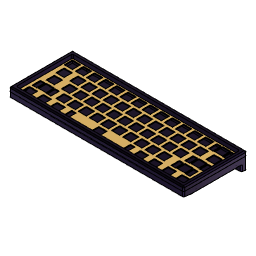
Anatidae60 v9 (Autodesk Fusion 360 design; units mm, degrees)
Autodesk Fusion 360 part; units mm, degrees
note: some values were not read from the file. Chosen so that the rebuilt part matches the saved one: which face or edge a step refers to; that a step has no effect; how an offset face is resized.
(part 1 of 2)
sketch "Sketch1" plane through (0, 0, 0) normal (0, 0, 1) x (1, 0, 0)
  line L0 (193.687761, 24.152837) -> (179.687761, 24.152837)
  line L1 (0.950846, 97.826737) -> (286.700761, 97.826737)
  line L2 (160.637761, 38.152237) -> (174.637761, 38.152237)
  line L3 (196.356761, 5.102877) -> (196.356761, 19.102337)
  line L4 (150.824761, 95.302337) -> (150.824761, 81.303037)
  line L5 (210.355761, 5.102877) -> (196.356761, 5.102877)
  line L6 (124.917761, 9.803347) -> (124.917761, 5.102877)
  line L7 (93.674761, 95.302337) -> (93.674761, 81.303037)
  line L8 (138.918761, 14.401837) -> (138.918761, 19.102337)
  line L9 (67.481061, 19.102337) -> (67.481061, 5.102877)
  line L10 (210.355761, 19.102337) -> (210.355761, 5.102877)
  line L11 (98.437261, 38.152237) -> (98.437261, 24.152837)
  line L12 (43.668561, 19.102337) -> (43.668561, 5.102877)
  line L13 (146.062761, 43.203037) -> (132.062761, 43.203037)
  line L14 (136.537761, 38.152237) -> (136.537761, 24.152837)
  line L15 (51.100461, 62.253037) -> (51.100461, 76.252337)
  line L16 (150.824761, 81.303037) -> (136.825761, 81.303037)
  line L17 (3.475411, 95.302337) -> (17.474961, 95.302337)
  line L18 (10.617791, 43.203037) -> (10.617791, 57.202337)
  line L19 (220.167761, 5.102877) -> (220.167761, 19.102337)
  line L20 (286.700761, 97.826737) -> (286.700761, 2.57693)
  line L21 (46.337961, 38.152237) -> (60.337261, 38.152237)
  line L22 (241.312761, 43.203037) -> (227.312761, 43.203037)
  line L23 (198.737761, 38.152237) -> (212.737761, 38.152237)
  line L24 (79.675461, 95.302337) -> (93.674761, 95.302337)
  line L25 (124.917761, 19.102337) -> (124.917761, 14.401837)
  line L26 (103.487761, 38.152237) -> (117.487761, 38.152237)
  line L27 (243.981761, 5.102877) -> (243.981761, 19.102337)
  line L28 (65.387961, 24.152837) -> (65.387961, 38.152237)
  line L29 (29.381161, 38.152237) -> (15.381661, 38.152237)
  line L30 (113.012761, 57.202337) -> (127.012761, 57.202337)
  line L31 (98.724061, 81.303037) -> (98.724061, 95.302337)
  line L32 (107.962761, 43.203037) -> (93.962961, 43.203037)
  line L33 (41.575461, 81.303037) -> (41.575461, 95.302337)
  line L34 (146.350761, 76.252337) -> (160.349761, 76.252337)
  line L35 (74.624761, 95.302337) -> (74.624761, 81.303037)
  line L36 (122.537761, 24.152837) -> (122.537761, 38.152237)
  line L37 (117.487761, 24.152837) -> (103.487761, 24.152837)
  line L38 (17.474961, 95.302337) -> (17.474961, 81.303037)
  line L39 (79.387261, 24.152837) -> (65.387961, 24.152837)
  line L40 (265.412761, 62.253037) -> (265.412761, 76.252337)
  line L41 (55.574761, 81.303037) -> (41.575461, 81.303037)
  line L42 (55.862961, 43.203037) -> (55.862961, 57.202337)
  line L43 (217.787761, 38.152237) -> (231.787761, 38.152237)
  line L44 (29.667761, 19.102337) -> (43.668561, 19.102337)
  line L45 (132.062761, 43.203037) -> (132.062761, 57.202337)
  line L46 (5.856671, 5.102877) -> (5.856671, 19.102337)
  line L47 (36.812961, 57.202337) -> (50.812261, 57.202337)
  line L48 (138.918761, 19.102337) -> (124.917761, 19.102337)
  line L49 (19.856161, 5.102877) -> (5.856671, 5.102877)
  line L50 (253.505761, 24.152837) -> (267.505761, 24.152837)
  line L51 (8.237921, 76.252337) -> (22.237461, 76.252337)
  line L52 (19.856161, 19.102337) -> (19.856161, 5.102877)
  line L53 (60.337261, 24.152837) -> (46.337961, 24.152837)
  line L54 (53.481761, 19.102337) -> (67.481061, 19.102337)
  line L55 (117.773761, 81.303037) -> (117.773761, 95.302337)
  line L56 (65.387961, 38.152237) -> (79.387261, 38.152237)
  line L57 (88.912261, 57.202337) -> (88.912261, 43.203037)
  line L58 (193.687761, 38.152237) -> (193.687761, 24.152837)
  line L59 (257.980761, 5.102877) -> (243.981761, 5.102877)
  line L60 (174.637761, 24.152837) -> (160.637761, 24.152837)
  line L61 (286.700761, 2.57693) -> (0.950846, 2.57693)
  line L62 (179.687761, 38.152237) -> (193.687761, 38.152237)
  line L63 (43.668561, 5.102877) -> (29.667761, 5.102877)
  line L64 (65.099761, 62.253037) -> (51.100461, 62.253037)
  line L65 (15.381661, 38.152237) -> (15.381661, 33.451837)
  line L66 (8.237921, 62.253037) -> (8.237921, 76.252337)
  line L67 (50.812261, 43.203037) -> (36.812961, 43.203037)
  line L68 (165.112761, 43.203037) -> (151.112761, 43.203037)
  line L69 (131.774761, 81.303037) -> (117.773761, 81.303037)
  line L70 (257.980761, 19.102337) -> (257.980761, 5.102877)
  line L71 (122.537761, 38.152237) -> (136.537761, 38.152237)
  line L72 (117.487761, 38.152237) -> (117.487761, 24.152837)
  line L73 (136.537761, 24.152837) -> (122.537761, 24.152837)
  line L74 (74.912961, 57.202337) -> (88.912261, 57.202337)
  line L75 (281.793761, 5.102877) -> (267.792761, 5.102877)
  line L76 (60.337261, 38.152237) -> (60.337261, 24.152837)
  line L77 (231.787761, 38.152237) -> (231.787761, 24.152837)
  line L78 (70.150461, 62.253037) -> (70.150461, 76.252337)
  line L79 (231.787761, 24.152837) -> (217.787761, 24.152837)
  line L80 (69.862261, 43.203037) -> (55.862961, 43.203037)
  line L81 (107.962761, 57.202337) -> (107.962761, 43.203037)
  line L82 (3.475411, 81.303037) -> (3.475411, 95.302337)
  line L83 (234.168761, 19.102337) -> (234.168761, 5.102877)
  line L84 (267.505761, 38.152237) -> (253.505761, 38.152237)
  line L85 (84.149761, 76.252337) -> (84.149761, 62.253037)
  line L86 (196.356761, 19.102337) -> (210.355761, 19.102337)
  line L87 (29.381161, 24.152837) -> (29.381161, 28.851937)
  line L88 (132.062761, 57.202337) -> (146.062761, 57.202337)
  line L89 (79.675461, 81.303037) -> (79.675461, 95.302337)
  line L90 (198.737761, 24.152837) -> (198.737761, 38.152237)
  line L91 (17.474961, 81.303037) -> (3.475411, 81.303037)
  line L92 (89.200461, 76.252337) -> (103.199761, 76.252337)
  line L93 (127.300761, 62.253037) -> (127.300761, 76.252337)
  line L94 (174.637761, 38.152237) -> (174.637761, 24.152837)
  line L95 (127.300761, 76.252337) -> (141.299761, 76.252337)
  line L96 (212.737761, 24.152837) -> (198.737761, 24.152837)
  line L97 (141.587761, 38.152237) -> (155.587761, 38.152237)
  line L98 (203.212761, 43.203037) -> (189.212761, 43.203037)
  line L99 (67.481061, 5.102877) -> (53.481761, 5.102877)
  line L100 (141.587761, 24.152837) -> (141.587761, 38.152237)
  line L101 (234.168761, 5.102877) -> (220.167761, 5.102877)
  line L102 (179.687761, 24.152837) -> (179.687761, 38.152237)
  line L103 (217.787761, 24.152837) -> (217.787761, 38.152237)
  line L104 (117.773761, 95.302337) -> (131.774761, 95.302337)
  line L105 (222.262761, 43.203037) -> (208.262761, 43.203037)
  line L106 (32.050461, 76.252337) -> (46.049761, 76.252337)
  line L107 (93.962961, 57.202337) -> (107.962761, 57.202337)
  line L108 (103.487761, 24.152837) -> (103.487761, 38.152237)
  line L109 (84.437961, 38.152237) -> (98.437261, 38.152237)
  line L110 (212.737761, 38.152237) -> (212.737761, 24.152837)
  line L111 (127.012761, 57.202337) -> (127.012761, 43.203037)
  line L112 (151.112761, 43.203037) -> (151.112761, 57.202337)
  line L113 (36.524761, 81.303037) -> (22.525461, 81.303037)
  line L114 (36.524761, 95.302337) -> (36.524761, 81.303037)
  line L115 (127.012761, 43.203037) -> (113.012761, 43.203037)
  line L116 (151.112761, 57.202337) -> (165.112761, 57.202337)
  line L117 (50.812261, 57.202337) -> (50.812261, 43.203037)
  line L118 (5.856671, 19.102337) -> (19.856161, 19.102337)
  line L119 (136.825761, 95.302337) -> (150.824761, 95.302337)
  line L120 (53.481761, 5.102877) -> (53.481761, 19.102337)
  line L121 (108.250761, 76.252337) -> (122.249761, 76.252337)
  line L122 (253.505761, 28.851937) -> (253.505761, 24.152837)
  line L123 (60.625461, 95.302337) -> (74.624761, 95.302337)
  line L124 (46.337961, 24.152837) -> (46.337961, 38.152237)
  line L125 (60.625461, 81.303037) -> (60.625461, 95.302337)
  line L126 (15.381661, 24.152837) -> (29.381161, 24.152837)
  line L127 (74.624761, 81.303037) -> (60.625461, 81.303037)
  line L128 (41.575461, 95.302337) -> (55.574761, 95.302337)
  line L129 (122.249761, 62.253037) -> (108.250761, 62.253037)
  line L130 (29.667761, 5.102877) -> (29.667761, 19.102337)
  line L131 (103.199761, 76.252337) -> (103.199761, 62.253037)
  line L132 (220.167761, 19.102337) -> (234.168761, 19.102337)
  line L133 (112.724761, 95.302337) -> (112.724761, 81.303037)
  line L134 (79.387261, 38.152237) -> (79.387261, 24.152837)
  line L135 (88.912261, 43.203037) -> (74.912961, 43.203037)
  line L136 (84.437961, 24.152837) -> (84.437961, 38.152237)
  line L137 (22.525461, 81.303037) -> (22.525461, 95.302337)
  line L138 (138.918761, 5.102877) -> (138.918761, 9.803347)
  line L139 (260.650761, 81.303037) -> (274.649761, 81.303037)
  line L140 (98.437261, 24.152837) -> (84.437961, 24.152837)
  line L141 (55.574761, 95.302337) -> (55.574761, 81.303037)
  line L142 (70.150461, 76.252337) -> (84.149761, 76.252337)
  line L143 (32.050461, 62.253037) -> (32.050461, 76.252337)
  line L144 (22.237461, 76.252337) -> (22.237461, 62.253037)
  line L145 (217.499761, 76.252337) -> (217.499761, 62.253037)
  line L146 (69.862261, 57.202337) -> (69.862261, 43.203037)
  line L147 (255.599761, 62.253037) -> (241.600761, 62.253037)
  line L148 (93.674761, 81.303037) -> (79.675461, 81.303037)
  line L149 (122.249761, 76.252337) -> (122.249761, 62.253037)
  line L150 (281.793761, 19.102337) -> (281.793761, 5.102877)
  line L151 (155.875761, 81.303037) -> (155.875761, 95.302337)
  line L152 (22.237461, 62.253037) -> (8.237921, 62.253037)
  line L153 (131.774761, 95.302337) -> (131.774761, 81.303037)
  line L154 (46.049761, 62.253037) -> (32.050461, 62.253037)
  line L155 (46.049761, 76.252337) -> (46.049761, 62.253037)
  line L156 (89.200461, 62.253037) -> (89.200461, 76.252337)
  line L157 (55.862961, 57.202337) -> (69.862261, 57.202337)
  line L158 (10.617791, 57.202337) -> (24.618661, 57.202337)
  line L159 (103.199761, 62.253037) -> (89.200461, 62.253037)
  line L160 (279.412761, 76.252337) -> (279.412761, 62.253037)
  line L161 (22.525461, 95.302337) -> (36.524761, 95.302337)
  line L162 (141.299761, 62.253037) -> (127.300761, 62.253037)
  line L163 (243.981761, 19.102337) -> (257.980761, 19.102337)
  line L164 (24.618661, 57.202337) -> (24.618661, 43.203037)
  line L165 (74.912961, 43.203037) -> (74.912961, 57.202337)
  line L166 (98.724061, 95.302337) -> (112.724761, 95.302337)
  line L167 (113.012761, 43.203037) -> (113.012761, 57.202337)
  line L168 (155.587761, 24.152837) -> (141.587761, 24.152837)
  line L169 (146.062761, 57.202337) -> (146.062761, 43.203037)
  line L170 (65.099761, 76.252337) -> (65.099761, 62.253037)
  line L171 (24.618661, 43.203037) -> (10.617791, 43.203037)
  line L172 (136.825761, 81.303037) -> (136.825761, 95.302337)
  line L173 (267.505761, 24.152837) -> (267.505761, 28.851937)
  line L174 (36.812961, 43.203037) -> (36.812961, 57.202337)
  line L175 (93.962961, 43.203037) -> (93.962961, 57.202337)
  line L176 (51.100461, 76.252337) -> (65.099761, 76.252337)
  line L177 (170.162761, 57.202337) -> (184.162761, 57.202337)
  line L178 (193.975761, 81.303037) -> (193.975761, 95.302337)
  line L179 (84.149761, 62.253037) -> (70.150461, 62.253037)
  line L180 (160.349761, 76.252337) -> (160.349761, 62.253037)
  line L181 (189.212761, 57.202337) -> (203.212761, 57.202337)
  line L182 (213.025761, 81.303037) -> (213.025761, 95.302337)
  line L183 (203.500761, 62.253037) -> (203.500761, 76.252337)
  line L184 (155.587761, 38.152237) -> (155.587761, 24.152837)
  line L185 (174.925761, 81.303037) -> (174.925761, 95.302337)
  line L186 (267.792761, 5.102877) -> (267.792761, 19.102337)
  line L187 (255.599761, 76.252337) -> (255.599761, 62.253037)
  line L188 (160.637761, 24.152837) -> (160.637761, 38.152237)
  line L189 (108.250761, 62.253037) -> (108.250761, 76.252337)
  line L190 (184.450761, 76.252337) -> (198.449761, 76.252337)
  line L191 (160.349761, 62.253037) -> (146.350761, 62.253037)
  line L192 (267.505761, 33.451837) -> (267.505761, 38.152237)
  line L193 (165.112761, 57.202337) -> (165.112761, 43.203037)
  line L194 (141.299761, 76.252337) -> (141.299761, 62.253037)
  line L195 (267.792761, 19.102337) -> (281.793761, 19.102337)
  line L196 (274.649761, 95.302337) -> (260.650761, 95.302337)
  line L197 (124.917761, 5.102877) -> (138.918761, 5.102877)
  line L198 (232.075761, 95.302337) -> (246.074761, 95.302337)
  line L199 (146.350761, 62.253037) -> (146.350761, 76.252337)
  line L200 (112.724761, 81.303037) -> (98.724061, 81.303037)
  line L201 (227.312761, 43.203037) -> (227.312761, 57.202337)
  line L202 (29.381161, 33.451837) -> (29.381161, 38.152237)
  line L203 (193.975761, 95.302337) -> (207.974761, 95.302337)
  line L204 (272.268761, 57.202337) -> (258.267761, 57.202337)
  line L205 (207.974761, 81.303037) -> (193.975761, 81.303037)
  line L206 (272.268761, 43.203037) -> (272.268761, 47.902037)
  line L207 (165.400761, 62.253037) -> (165.400761, 76.252337)
  line L208 (184.450761, 62.253037) -> (184.450761, 76.252337)
  line L209 (246.074761, 81.303037) -> (232.075761, 81.303037)
  line L210 (15.381661, 28.851937) -> (15.381661, 24.152837)
  line L211 (222.550761, 76.252337) -> (236.549761, 76.252337)
  line L212 (207.974761, 95.302337) -> (207.974761, 81.303037)
  line L213 (253.505761, 38.152237) -> (253.505761, 33.451837)
  line L214 (222.550761, 62.253037) -> (222.550761, 76.252337)
  line L215 (246.074761, 95.302337) -> (246.074761, 81.303037)
  line L216 (274.649761, 90.601837) -> (274.649761, 95.302337)
  line L217 (274.649761, 81.303037) -> (274.649761, 86.002037)
  line L218 (208.262761, 43.203037) -> (208.262761, 57.202337)
  line L219 (179.399761, 62.253037) -> (165.400761, 62.253037)
  line L220 (217.499761, 62.253037) -> (203.500761, 62.253037)
  line L221 (203.212761, 57.202337) -> (203.212761, 43.203037)
  line L222 (227.024761, 81.303037) -> (213.025761, 81.303037)
  line L223 (236.549761, 62.253037) -> (222.550761, 62.253037)
  line L224 (169.874761, 95.302337) -> (169.874761, 81.303037)
  line L225 (227.024761, 95.302337) -> (227.024761, 81.303037)
  line L226 (241.600761, 76.252337) -> (255.599761, 76.252337)
  line L227 (236.549761, 76.252337) -> (236.549761, 62.253037)
  line L228 (232.075761, 81.303037) -> (232.075761, 95.302337)
  line L229 (241.600761, 62.253037) -> (241.600761, 76.252337)
  line L230 (258.267761, 43.203037) -> (272.268761, 43.203037)
  line L231 (188.924761, 81.303037) -> (174.925761, 81.303037)
  line L232 (188.924761, 95.302337) -> (188.924761, 81.303037)
  line L233 (170.162761, 43.203037) -> (170.162761, 57.202337)
  line L234 (179.399761, 76.252337) -> (179.399761, 62.253037)
  line L235 (203.500761, 76.252337) -> (217.499761, 76.252337)
  line L236 (241.312761, 57.202337) -> (241.312761, 43.203037)
  line L237 (169.874761, 81.303037) -> (155.875761, 81.303037)
  line L238 (227.312761, 57.202337) -> (241.312761, 57.202337)
  line L239 (279.412761, 62.253037) -> (265.412761, 62.253037)
  line L240 (222.262761, 57.202337) -> (222.262761, 43.203037)
  line L241 (258.267761, 57.202337) -> (258.267761, 52.501837)
  line L242 (198.449761, 76.252337) -> (198.449761, 62.253037)
  line L243 (208.262761, 57.202337) -> (222.262761, 57.202337)
  line L244 (213.025761, 95.302337) -> (227.024761, 95.302337)
  line L245 (265.412761, 76.252337) -> (279.412761, 76.252337)
  line L246 (272.268761, 52.501837) -> (272.268761, 57.202337)
  line L247 (155.875761, 95.302337) -> (169.874761, 95.302337)
  line L248 (198.449761, 62.253037) -> (184.450761, 62.253037)
  line L249 (258.267761, 47.902037) -> (258.267761, 43.203037)
  line L250 (184.162761, 43.203037) -> (170.162761, 43.203037)
  line L251 (0.950846, 2.57693) -> (0.950846, 97.826737)
  line L252 (184.162761, 57.202337) -> (184.162761, 43.203037)
  line L253 (189.212761, 43.203037) -> (189.212761, 57.202337)
  line L254 (165.400761, 76.252337) -> (179.399761, 76.252337)
  line L255 (174.925761, 95.302337) -> (188.924761, 95.302337)
  line L256 (13.856161, 37.604037) -> (6.279122, 37.604037)
  line L257 (6.279122, 37.604037) -> (6.279122, 23.409352)
  line L258 (6.279122, 23.409352) -> (13.856161, 23.409352)
  line L259 (13.856161, 23.409352) -> (13.856161, 37.604037)
  line L260 (30.906661, 37.604037) -> (38.489856, 37.604037)
  line L261 (38.489856, 37.604037) -> (38.489856, 23.409352)
  line L262 (38.489856, 23.409352) -> (30.906661, 23.409352)
  line L263 (30.906661, 23.409352) -> (30.906661, 37.604037)
  line L264 (15.381661, 33.451837) -> (15.381661, 28.851937)
  line L265 (29.381161, 33.451837) -> (29.381161, 28.851937)
  line L266 (253.505761, 33.451837) -> (253.505761, 28.851937)
  line L267 (267.505761, 33.451837) -> (267.505761, 28.851937)
  line L268 (258.267761, 52.501837) -> (258.267761, 47.902037)
  line L269 (272.268761, 52.501837) -> (272.268761, 47.902037)
  line L270 (260.650761, 95.302337) -> (260.650761, 81.303037)
  line L271 (274.649761, 90.601837) -> (274.649761, 86.002037)
  line L272 (30.906661, 23.409352) -> (30.906661, 37.604037)
  line L273 (38.489856, 37.604037) -> (38.489856, 23.409352)
  line L274 (38.489856, 23.409352) -> (30.906661, 23.409352)
  line L275 (30.906661, 37.604037) -> (38.489856, 37.604037)
  line L276 (6.279122, 37.604037) -> (6.279122, 23.409352)
  line L277 (13.856161, 37.604037) -> (6.279122, 37.604037)
  line L278 (13.856161, 23.409352) -> (13.856161, 37.604037)
  line L279 (6.279122, 23.409352) -> (13.856161, 23.409352)
  line L280 (6.279122, 37.604037) -> (6.279122, 23.409352)
  line L281 (13.856161, 37.604037) -> (6.279122, 37.604037)
  line L282 (13.856161, 23.409352) -> (13.856161, 37.604037)
  line L283 (6.279122, 23.409352) -> (13.856161, 23.409352)
  line L284 (273.794161, 42.459352) -> (273.794161, 56.654037)
  line L285 (273.794161, 56.654037) -> (281.377356, 56.654037)
  line L286 (281.377356, 42.459352) -> (273.794161, 42.459352)
  line L287 (281.377356, 42.459352) -> (273.794161, 42.459352)
  line L288 (273.794161, 56.654037) -> (281.377356, 56.654037)
  line L289 (281.377356, 56.654037) -> (281.377356, 42.459352)
  line L290 (273.794161, 42.459352) -> (273.794161, 56.654037)
  line L291 (281.377356, 56.654037) -> (281.377356, 42.459352)
  line L292 (249.166622, 56.654037) -> (249.166622, 42.459352)
  line L293 (256.743661, 56.654037) -> (249.166622, 56.654037)
  line L294 (256.743661, 42.459352) -> (256.743661, 56.654037)
  line L295 (249.166622, 42.459352) -> (256.743661, 42.459352)
  line L296 (269.031661, 23.409352) -> (269.031661, 37.604037)
  line L297 (269.031661, 37.604037) -> (276.614856, 37.604037)
  line L298 (276.614856, 23.409352) -> (269.031661, 23.409352)
  line L299 (276.614856, 23.409352) -> (269.031661, 23.409352)
  line L300 (269.031661, 37.604037) -> (276.614856, 37.604037)
  line L301 (276.614856, 37.604037) -> (276.614856, 23.409352)
  line L302 (269.031661, 23.409352) -> (269.031661, 37.604037)
  line L303 (276.614856, 37.604037) -> (276.614856, 23.409352)
  line L304 (244.404122, 37.604037) -> (244.404122, 23.409352)
  line L305 (251.981161, 37.604037) -> (244.404122, 37.604037)
  line L306 (251.981161, 23.409352) -> (251.981161, 37.604037)
  line L307 (244.404122, 23.409352) -> (251.981161, 23.409352)
  line L308 (30.906661, 23.409352) -> (30.906661, 37.604037)
  line L309 (30.906661, 37.604037) -> (38.489856, 37.604037)
  line L310 (38.489856, 23.409352) -> (30.906661, 23.409352)
  line L311 (38.489856, 23.409352) -> (30.906661, 23.409352)
  line L312 (30.906661, 37.604037) -> (38.489856, 37.604037)
  line L313 (38.489856, 37.604037) -> (38.489856, 23.409352)
  line L314 (30.906661, 23.409352) -> (30.906661, 37.604037)
  line L315 (38.489856, 37.604037) -> (38.489856, 23.409352)
  line L316 (6.279122, 37.604037) -> (6.279122, 23.409352)
  line L317 (13.856161, 37.604037) -> (6.279122, 37.604037)
  line L318 (13.856161, 23.409352) -> (13.856161, 37.604037)
  line L319 (6.279122, 23.409352) -> (13.856161, 23.409352)
  line L320 (13.856161, 23.409352) -> (13.856161, 37.604037)
  line L321 (13.856161, 23.409352) -> (13.856161, 37.604037)
  line L322 (6.279122, 37.604037) -> (6.279122, 23.409352)
  line L323 (6.279122, 37.604037) -> (6.279122, 23.409352)
  line L324 (6.279122, 37.604037) -> (6.279122, 23.409352)
  line L325 (6.279122, 37.604037) -> (6.279122, 23.409352)
  line L326 (13.856161, 23.409352) -> (13.856161, 37.604037)
  line L327 (13.856161, 23.409352) -> (13.856161, 37.604037)
  line L328 (13.856161, 37.604037) -> (6.279122, 37.604037)
  line L329 (13.856161, 37.604037) -> (6.279122, 37.604037)
  line L330 (6.279122, 23.409352) -> (13.856161, 23.409352)
  line L331 (13.856161, 37.604037) -> (6.279122, 37.604037)
  line L332 (6.279122, 23.409352) -> (13.856161, 23.409352)
  line L333 (6.279122, 23.409352) -> (13.856161, 23.409352)
  line L334 (6.279122, 23.409352) -> (13.856161, 23.409352)
  line L335 (13.856161, 37.604037) -> (6.279122, 37.604037)
  line L336 (30.906661, 23.409352) -> (30.906661, 37.604037)
  line L337 (30.906661, 37.604037) -> (38.489856, 37.604037)
  line L338 (38.489856, 37.604037) -> (38.489856, 23.409352)
  line L339 (38.489856, 23.409352) -> (30.906661, 23.409352)
  line L340 (259.124911, 80.559352) -> (259.124911, 94.754037)
  line L341 (259.124911, 80.559352) -> (259.124911, 94.754037)
  line L342 (251.547872, 94.754037) -> (251.547872, 80.559352)
  line L343 (251.547872, 94.754037) -> (251.547872, 80.559352)
  line L344 (251.547872, 94.754037) -> (251.547872, 80.559352)
  line L345 (251.547872, 94.754037) -> (251.547872, 80.559352)
  line L346 (259.124911, 80.559352) -> (259.124911, 94.754037)
  line L347 (259.124911, 80.559352) -> (259.124911, 94.754037)
  line L348 (259.124911, 94.754037) -> (251.547872, 94.754037)
  line L349 (259.124911, 94.754037) -> (251.547872, 94.754037)
  line L350 (251.547872, 80.559352) -> (259.124911, 80.559352)
  line L351 (259.124911, 94.754037) -> (251.547872, 94.754037)
  line L352 (251.547872, 80.559352) -> (259.124911, 80.559352)
  line L353 (251.547872, 80.559352) -> (259.124911, 80.559352)
  line L354 (251.547872, 80.559352) -> (259.124911, 80.559352)
  line L355 (259.124911, 94.754037) -> (251.547872, 94.754037)
  line L356 (276.175411, 80.559352) -> (276.175411, 94.754037)
  line L357 (276.175411, 94.754037) -> (283.758606, 94.754037)
  line L358 (283.758606, 94.754037) -> (283.758606, 80.559352)
  line L359 (283.758606, 80.559352) -> (276.175411, 80.559352)
  line L360 (85.293861, 4.350514) -> (77.718661, 4.350514)
  line L361 (124.917761, 14.401837) -> (124.917761, 9.803347)
  line L362 (186.117761, 4.337226) -> (178.542761, 4.337226)
  line L363 (138.918761, 14.401837) -> (138.918761, 9.803347)
  line L364 (85.293861, 19.85467) -> (77.718661, 19.85467)
  line L365 (186.117761, 19.867958) -> (178.542761, 19.867958)
  line L366 (77.718661, 19.85467) -> (77.718661, 4.350514)
  line L367 (186.117761, 19.867958) -> (186.117761, 4.337226)
  line L368 (178.542761, 4.337226) -> (178.542761, 19.867958)
  line L369 (85.293861, 4.350514) -> (85.293861, 19.85467)
  line L370 (0.475846, 98.301737) -> (287.175761, 98.301737)
  line L371 (287.175761, 98.301737) -> (287.175761, 2.10193)
  line L372 (287.175761, 2.10193) -> (0.475846, 2.10193)
  line L373 (0.475846, 2.10193) -> (0.475846, 98.301737)
  line L374 (293.175761, -3.89807) -> (-5.524154, -3.89807)
  line L375 (-5.524154, -3.89807) -> (-5.524154, 104.301737)
  line L376 (-5.524154, 104.301737) -> (293.175761, 104.301737)
  line L377 (293.175761, 104.301737) -> (293.175761, -3.89807)
  dimension "d1" = -0.475
  dimension "d2" = -6.475
  constraint horizontal L256
  constraint horizontal L258
  constraint vertical L259
  constraint horizontal L260
  constraint vertical L261
  constraint horizontal L262
  constraint vertical L263
  constraint parallel L210 L264
  constraint parallel L213 L266
  constraint parallel L173 L267
  constraint parallel L249 L268
  constraint parallel L206 L269
  constraint perpendicular L139 L270
  constraint parallel L217 L271
  constraint horizontal L277
  constraint horizontal L279
  constraint vertical L278
  constraint horizontal L275
  constraint vertical L273
  constraint horizontal L274
  constraint vertical L272
  constraint horizontal L281
  constraint horizontal L283
  constraint vertical L282
  constraint horizontal L293
  constraint vertical L294
  constraint horizontal L288
  constraint vertical L289
  constraint horizontal L286
  constraint vertical L290
  constraint horizontal L295
  constraint horizontal L285
  constraint vertical L291
  constraint horizontal L287
  constraint vertical L284
  constraint horizontal L305
  constraint vertical L306
  constraint horizontal L300
  constraint vertical L301
  constraint horizontal L298
  constraint vertical L302
  constraint horizontal L307
  constraint horizontal L297
  constraint vertical L303
  constraint horizontal L299
  constraint vertical L296
  constraint horizontal L317
  constraint vertical L318
  constraint horizontal L312
  constraint vertical L313
  constraint horizontal L310
  constraint vertical L314
  constraint horizontal L319
  constraint horizontal L309
  constraint vertical L315
  constraint horizontal L311
  constraint vertical L308
  constraint horizontal L329
  constraint horizontal L333
  constraint vertical L320
  constraint horizontal L337
  constraint horizontal L339
  constraint vertical L336
  constraint horizontal L331
  constraint horizontal L332
  constraint vertical L327
  constraint vertical L338
  constraint horizontal L328
  constraint horizontal L330
  constraint vertical L326
  constraint horizontal L335
  constraint vertical L321
  constraint horizontal L334
  constraint horizontal L349
  constraint horizontal L353
  constraint vertical L340
  constraint horizontal L357
  constraint horizontal L359
  constraint vertical L356
  constraint horizontal L351
  constraint horizontal L352
  constraint vertical L347
  constraint vertical L358
  constraint horizontal L348
  constraint horizontal L350
  constraint vertical L346
  constraint horizontal L355
  constraint vertical L341
  constraint horizontal L354
  constraint horizontal L360
  constraint perpendicular L48 L361
  constraint horizontal L362
  constraint parallel L138 L363
  constraint perpendicular L360 L366
  constraint perpendicular L362 L367
  constraint perpendicular L365 L368
  constraint perpendicular L364 L369
extrude "Extrude5" add sketch "Sketch1" along normal blind 1.5 contours L1 L20 L61 L251 picked at (159.366428, 11.197647) makes body 1
extrude "Extrude1" add sketch "Sketch1" along normal blind 7.5 separate body contours L374 L375 L376 L377 picked at (191.609123, -1.89807) makes body 2
sketch "Sketch4" plane through (293.175761, 0, 0) normal (1, 0, 0) x (0, 1, 0)
  line L0 (-3.89807, 0) -> (104.301737, 0)
  line L1 (104.301737, 0) -> (104.301737, 7.5)
  line L2 (104.301737, 7.5) -> (-3.89807, 7.5)
  line L3 (-3.89807, 7.5) -> (-3.89807, 0)
  line L4 (-3.89807, 0) -> (-3.89807, -7.75)
  line L5 (-3.89807, -7.75) -> (104.301737, -20.967998)
  line L6 (104.301737, -20.967998) -> (104.301737, 0)
  dimension "d7" = 7.75
  constraint perpendicular L0 L4
  constraint perpendicular L0 L6
extrude "Extrude2" add sketch "Sketch4" against normal blind 350 separate body contours L0 L4 L5 L6 picked at (68.235135, -9.572666) makes body 3
sketch "Sketch5" plane through (0, -3.89807, 0) normal (0, -1, 0) x (1, 0, 0)
  line L0 (-5.524154, 0) -> (293.175761, 0)
  line L1 (293.175761, 0) -> (293.175761, 7.5)
  line L2 (293.175761, 7.5) -> (-5.524154, 7.5)
  line L3 (-5.524154, 7.5) -> (-5.524154, 0)
  line L4 (-5.524154, 7.5) -> (-64.000001, 7.5)
  line L5 (-64.000001, 7.5) -> (-64.000001, -35.000001)
  line L6 (-64.000001, -35.000001) -> (-5.524154, -35.000001)
  line L7 (-5.524154, -35.000001) -> (-5.524154, 7.5)
  constraint horizontal L4
  constraint vertical L5
  constraint horizontal L6
  constraint vertical L7
extrude "Extrude3" cut sketch "Sketch5" against normal blind 120 contours L3 L4 L5 L6 L7 picked at (-44.508052, -9.166667) bodies 3
extrude "Extrude4" cut sketch "Sketch1" against normal blind 4.2 contours L0 L58 L62 L102 | L1 L20 L61 L251 | L2 L60 L94 L188 | L3 L5 L10 L86 | L4 L16 L119 L172 | L6 L8 L25 L48 L138 L197 L361 L363 | L7 L24 L89 L148 | L9 L54 L99 L120 | L11 L109 L136 L140 | L12 L44 L63 L130 | L13 L45 L88 L169 | L14 L36 L71 L73 | L15 L64 L170 L176 | L17 L38 L82 L91 | L18 L158 L164 L171 | L19 L83 L101 L132 | L21 L53 L76 L124 | L22 L201 L236 L238 | L23 L90 L96 L110 | L26 L37 L72 L108 | L27 L59 L70 L163 | L28 L39 L56 L134 | L29 L65 L87 L126 L202 L210 L264 L265 | L30 L111 L115 L167 | L31 L133 L166 L200 | L32 L81 L107 L175 | L33 L41 L128 L141 | L34 L180 L191 L199 | L35 L123 L125 L127 | L40 L160 L239 L245 | L42 L80 L146 L157 | L43 L77 L79 L103 | L46 L49 L52 L118 | L47 L67 L117 L174 | L50 L84 L122 L173 L192 L213 L266 L267 | L51 L66 L144 L152 | L55 L69 L104 L153 | L57 L74 L135 L165 | L68 L112 L116 L193 | L75 L150 L186 L195 | L78 L85 L142 L179 | L92 L131 L156 L159 | L93 L95 L162 L194 | L97 L100 L168 L184 | L98 L181 L221 L253 | L105 L218 L240 L243 | L106 L143 L154 L155 | L113 L114 L137 L161 | L121 L129 L149 L189 | L139 L196 L216 L217 L270 L271 | L145 L183 L220 L235 | L147 L187 L226 L229 | L151 L224 L237 L247 | L177 L233 L250 L252 | L178 L203 L205 L212 | L182 L222 L225 L244 | L185 L231 L232 L255 | L190 L208 L242 L248 | L198 L209 L215 L228 | L204 L206 L230 L241 L246 L249 L268 L269 | L207 L219 L234 L254 | L211 L214 L223 L227 | L256 L257 L258 L259 L276 L277 L278 L279 L280 L281 L282 L283 L316 L317 L318 L319 L320 L321 L322 L323 L324 L325 L326 L327 L328 L329 L330 L331 L332 L333 L334 L335 | L260 L261 L262 L263 L272 L273 L274 L275 L308 L309 L310 L311 L312 L313 L314 L315 L336 L337 L338 L339 | L284 L285 L286 L287 L288 L289 L290 L291 | L292 L293 L294 L295 | L296 L297 L298 L299 L300 L301 L302 L303 | L304 L305 L306 L307 | L340 L341 L342 L343 L344 L345 L346 L347 L348 L349 L350 L351 L352 L353 L354 L355 | L356 L357 L358 L359 | L360 L364 L366 L369 | L362 L365 L367 L368 | L370 L371 L372 L373 picked at (184.354428, 28.819304) picked at (159.366428, 11.197647) picked at (165.304428, 28.819304) picked at (205.689428, 9.769364) picked at (141.492095, 85.96947) picked at (129.584761, 17.535504) picked at (84.341895, 90.635904) picked at (58.148195, 14.43585) picked at (89.104395, 33.48577) picked at (39.001628, 9.769364) picked at (141.396095, 47.86947) picked at (127.204428, 33.48577) picked at (55.766895, 71.585904) picked at (8.141928, 85.96947) picked at (15.284748, 47.86947) picked at (224.834761, 14.43585) picked at (51.004395, 28.819304) picked at (231.979428, 52.535904) picked at (208.071095, 33.48577) picked at (108.154428, 33.48577) picked at (248.648095, 9.769364) picked at (70.054395, 33.48577) picked at (20.048161, 36.585437) picked at (117.679428, 52.535904) picked at (103.390961, 85.96947) picked at (98.629561, 52.535904) picked at (46.241895, 90.635904) picked at (151.017095, 71.585904) picked at (65.291895, 90.635904) picked at (270.079428, 71.585904) picked at (60.529395, 47.86947) picked at (227.121095, 33.48577) picked at (10.523168, 14.43585) picked at (41.479395, 52.535904) picked at (258.172428, 36.585437) picked at (12.904435, 71.585904) picked at (122.440761, 85.96947) picked at (79.579395, 52.535904) picked at (160.446095, 47.86947) picked at (272.459761, 9.769364) picked at (74.816895, 66.91947) picked at (93.866895, 66.91947) picked at (131.967095, 66.91947) picked at (146.254428, 33.48577) picked at (198.546095, 47.86947) picked at (217.596095, 47.86947) picked at (41.383328, 71.585904) picked at (27.191895, 85.96947) picked at (112.917095, 71.585904) picked at (265.317095, 89.06907) picked at (208.167095, 71.585904) picked at (250.933428, 66.91947) picked at (160.542095, 85.96947) picked at (174.829428, 52.535904) picked at (198.642095, 85.96947) picked at (217.692095, 85.96947) picked at (179.592095, 85.96947) picked at (189.117095, 71.585904) picked at (236.742095, 85.96947) picked at (262.934761, 55.635504) picked at (170.067095, 71.585904) picked at (227.217095, 71.585904) picked at (8.804802, 32.872475) picked at (33.434393, 28.140914) picked at (278.849624, 47.190914) picked at (251.692302, 47.190914) picked at (271.559393, 32.872475) picked at (246.929802, 32.872475) picked at (256.599232, 85.290914) picked at (278.703143, 90.022475) picked at (82.768795, 9.518566) picked at (183.592761, 14.691047) picked at (96.200818, 2.260263) bodies 3
fillet "Fillet1" radius 2 8 edges at (293.175761, -3.89807, 3.75) (293.175761, 104.301737, 3.75) (-5.524154, -3.89807, 3.75) (-5.524154, 104.301737, 3.75) (293.175761, -3.89807, -3.875) (293.175761, 104.301737, -10.483999) (-5.524154, -3.89807, -3.875) (-5.524154, 104.301737, -10.483999) on bodies 2 3
chamfer "Chamfer1" distance 2 angle 45 8 edges at (292.589975, -3.312284, 7.5) (143.825804, -3.89807, 7.5) (-4.938368, -3.312284, 7.5) (-5.524154, 50.201833, 7.5) (-4.938368, 103.715951, 7.5) (143.825804, 104.301737, 7.5) (292.589975, 103.715951, 7.5) (293.175761, 50.201833, 7.5) on bodies 2
fillet "Fillet2" radius 2 4 edges at (0.475846, 98.301737, 3.75) (0.475846, 2.10193, 3.75) (287.175761, 2.10193, 3.75) (287.175761, 98.301737, 3.75) on bodies 2
fillet "Fillet3" radius 2 4 edges at (286.700761, 97.826737, 0.75) (286.700761, 2.57693, 0.75) (0.950846, 2.57693, 0.75) (0.950846, 97.826737, 0.75) on bodies 1
sketch "Sketch7" plane through (0, 0, 0) normal (0, 0, 1) x (-1, 0, 0)
  arc A0 (3.524154, -104.301737) -> (5.524154, -102.301737) centre (3.524154, -102.301737) ccw
  line L0 (5.524154, -102.301737) -> (5.524154, 1.89807)
  arc A1 (5.524154, 1.89807) -> (3.524154, 3.89807) centre (3.524154, 1.89807) ccw
  line L1 (3.524154, 3.89807) -> (-291.175761, 3.89807)
  arc A2 (-291.175761, 3.89807) -> (-293.175761, 1.89807) centre (-291.175761, 1.89807) ccw
  line L2 (-293.175761, 1.89807) -> (-293.175761, -102.301737)
  arc A3 (-293.175761, -102.301737) -> (-291.175761, -104.301737) centre (-291.175761, -102.301737) ccw
  line L3 (-291.175761, -104.301737) -> (3.524154, -104.301737)
  line L4 (-287.175761, -98.301737) -> (-287.175761, -2.10193)
  line L5 (-287.175761, -2.10193) -> (-0.475846, -2.10193)
  line L6 (-0.475846, -2.10193) -> (-0.475846, -98.301737)
  line L7 (-0.475846, -98.301737) -> (-287.175761, -98.301737)
  line L8 (-143.825804, -2.10193) -> (-63.825804, -2.10193)
  line L9 (-63.825804, -2.10193) -> (-63.825804, 2.99807)
  line L10 (-63.825804, 2.99807) -> (-143.825804, 2.99807)
  line L11 (-143.825804, 2.99807) -> (-143.825804, -2.10193)
  line L12 (-143.825804, -2.10193) -> (-223.825804, -2.10193)
  line L13 (-223.825804, -2.10193) -> (-223.825804, 2.99807)
  line L14 (-223.825804, 2.99807) -> (-143.825804, 2.99807)
  line L15 (-143.825804, 2.99807) -> (-143.825804, -2.10193)
  line L16 (-143.825804, -98.301737) -> (-63.825804, -98.301737)
  line L17 (-63.825804, -98.301737) -> (-63.825804, -103.401737)
  line L18 (-63.825804, -103.401737) -> (-143.825804, -103.401737)
  line L19 (-143.825804, -103.401737) -> (-143.825804, -98.301737)
  line L20 (-143.825804, -103.401737) -> (-223.825804, -103.401737)
  line L21 (-223.825804, -103.401737) -> (-223.825804, -98.301737)
  line L22 (-223.825804, -98.301737) -> (-143.825804, -98.301737)
  line L23 (-143.825804, -98.301737) -> (-143.825804, -103.401737)
  dimension "d24" = 80
  dimension "d25" = 5.1
  dimension "d26" = 80
  dimension "d27" = 5.1
  dimension "d28" = 80
  constraint horizontal L8
  constraint vertical L9
  constraint horizontal L10
  constraint vertical L11
  constraint horizontal L12
  constraint vertical L13
  constraint horizontal L14
  constraint vertical L15
  constraint horizontal L16
  constraint vertical L17
  constraint horizontal L18
  constraint vertical L19
  constraint horizontal L20
  constraint vertical L21
  constraint horizontal L22
  constraint vertical L23
extrude "Extrude6" cut sketch "Sketch7" against normal blind 2 contours L7 L19 L20 L21 L22 L23 | L5 L11 L12 L13 L14 L15 | L7 L16 L17 L18 L19 L23 | L5 L8 L9 L10 L11 L15 picked at (-197.159137, -100.001737) picked at (-170.49247, -0.40193) picked at (-117.159137, -100.001737) picked at (-117.159137, 1.29807) bodies 3
sketch "Sketch8" plane through (293.175761, 0, 0) normal (1, 0, 0) x (0, 1, 0)
  line L0 (102.301737, -20.723672) -> (102.301737, 0)
  line L1 (102.301737, 0) -> (-1.89807, 0)
  line L2 (-1.89807, 0) -> (-1.89807, -7.994326)
  line L3 (-1.89807, -7.994326) -> (102.301737, -20.723672)
  line L4 (10.048794, -9.453789) -> (95.000001, -9.453789)
  line L5 (95.000001, -9.453789) -> (95.000001, -19.831671)
  constraint perpendicular L4 L5
extrude "Extrude8" cut sketch "Sketch8" against normal blind 10 contours L3 L4 L5 picked at (66.682932, -12.913083) bodies 3
extrude "Extrude7" cut sketch "Sketch8" against normal blind 5 contours L3 L4 L5 picked at (66.682932, -12.913083) bodies 3
sketch "Sketch9" plane through (-5.524154, 0, 0) normal (-1, 0, 0) x (0, -1, 0)
  line L0 (-102.301737, 0) -> (-102.301737, -20.723672)
  line L1 (-102.301737, -20.723672) -> (1.89807, -7.994326)
  line L2 (1.89807, -7.994326) -> (1.89807, 0)
  line L3 (1.89807, 0) -> (-102.301737, 0)
sketch "Sketch10" plane through (-5.524154, 0, 0) normal (-1, 0, 0) x (0, -1, 0)
  line L0 (-10, -9.5) -> (-95.000001, -9.5)
  line L1 (-95.000001, -9.5) -> (-95.000001, -20)
  line L2 (-95.000001, -20) -> (-10, -9.5)
  constraint horizontal L0
  constraint perpendicular L0 L1
extrude "Extrude9" cut sketch "Sketch10" against normal blind 10 bodies 3
fillet "Fillet4" radius 2 4 edges at (293.175761, 95.000001, -14.64273) (-5.524154, 95.000001, -14.665836) (4.475846, 95.000001, -14.665836) (283.175761, 95.000001, -14.64273) on bodies 3
extrude "Extrude10" cut 1 faces at (96.042484, 34.168532, -4.2) along direction (0, 0, -1) blind 2 on bodies 3 bodies 3
sketch "Sketch11" plane through (0, 104.301737, 0) normal (0, 1, 0) x (-1, 0, 0)
  line L0 (3.524154, -20.967998) -> (3.524154, 0)
  line L1 (3.524154, 0) -> (-291.175761, 0)
  line L2 (-291.175761, 0) -> (-291.175761, -20.967998)
  line L3 (-291.175761, -20.967998) -> (3.524154, -20.967998)
  line L4 (-25.5, -2) -> (-25.5, -6)
  line L5 (-15.5, -2) -> (-15.5, -6)
  line L6 (-25.5, -6) -> (-15.5, -6)
  line L7 (-25.5, -1) -> (-15.5, -1)
  line L8 (-25.5, -1) -> (-25.5, -2)
  line L9 (-15.5, -1) -> (-15.5, -2)
  line L10 (-25.5, -1) -> (-15.5, -1)
  line L11 (-15.5, -1) -> (-15.5, -1.25)
  line L12 (-15.5, -1.25) -> (-25.5, -1.25)
  line L13 (-25.5, -1.25) -> (-25.5, -1)
  line L14 (-25.5, -1) -> (-25, -1)
  line L15 (-25, -1) -> (-25, -6)
  line L16 (-25, -6) -> (-25.5, -6)
  line L17 (-25.5, -6) -> (-25.5, -1)
  line L18 (-15.5, -1) -> (-16, -1)
  line L19 (-16, -1) -> (-16, -6)
  line L20 (-16, -6) -> (-15.5, -6)
  line L21 (-15.5, -6) -> (-15.5, -1)
  line L22 (-25.5, -6) -> (-15.5, -6)
  line L23 (-15.5, -6) -> (-15.5, -5.75)
  line L24 (-15.5, -5.75) -> (-25.5, -5.75)
  line L25 (-25.5, -5.75) -> (-25.5, -6)
  dimension "d47" = 4
  dimension "d48" = 4
  dimension "d49" = 0.25
  dimension "d50" = 0.5
  dimension "d51" = 0.5
  dimension "d52" = 0.25
  constraint perpendicular L1 L4
  constraint parallel L4 L8
  constraint parallel L5 L9
  constraint horizontal L10
  constraint vertical L11
  constraint horizontal L12
  constraint vertical L13
  constraint horizontal L14
  constraint vertical L15
  constraint horizontal L16
  constraint vertical L17
  constraint horizontal L18
  constraint vertical L19
  constraint horizontal L20
  constraint vertical L21
  constraint coincident L6 L19.end
  constraint horizontal L22
  constraint vertical L23
  constraint horizontal L24
  constraint vertical L25
  measures "d47" distance of L4.start L4.end
  measures "d48" distance of L5.start L5.end
  measures "d49" distance of L7.start L12.end
  measures "d50" distance of L7.start L14.end
  measures "d51" distance of L7.end L18.end
  measures "d52" distance of L4.end L24.end
extrude "Extrude11" cut sketch "Sketch11" against normal blind 9 contours L12 L15 L19 L24 picked at (-22, -2.75) bodies 3
fillet "Fillet5" radius 0.5 4 edges at (16, 101.301737, -1.25) (25, 101.301737, -1.25) (16, 101.301737, -5.75) (25, 101.301737, -5.75) on bodies 3
fillet "Fillet6" radius 0.4 8 edges at (25, 104.301737, -3.5) (24.853553, 104.301737, -5.603553) (20.5, 104.301737, -5.75) (16.146447, 104.301737, -5.603553) (16, 104.301737, -3.5) (16.146447, 104.301737, -1.396447) (20.5, 104.301737, -1.25) (24.853553, 104.301737, -1.396447) on bodies 3
sketch "Sketch12" plane through (0, 0, -9.453789) normal (0, 0, -1) x (1, 0, 0)
  arc A0 (283.175761, -93.000001) -> (285.175761, -95.000001) centre (285.175761, -93.000001) ccw
  line L0 (285.175761, -95.000001) -> (291.175761, -95.000001)
  arc A1 (293.175761, -97.000001) -> (291.175761, -95.000001) centre (291.175761, -97.000001) ccw
  line L1 (293.175761, -97.000001) -> (293.175761, -10.048794)
  line L2 (293.175761, -10.048794) -> (283.175761, -10.048794)
  line L3 (283.175761, -10.048794) -> (283.175761, -93.000001)
  circle A2 centre (0, -18) radius 3
  circle A3 centre (0, -87) radius 3
  circle A4 centre (288.175761, -18.048794) radius 3
  circle A5 centre (288.175761, -87.000001) radius 3
  dimension "d62" = 6
  dimension "d63" = 6
  dimension "d66" = 6
  dimension "d67" = 6
  measures "d62" diameter of A2
  measures "d63" diameter of A3
  measures "d66" diameter of A4
  measures "d67" diameter of A5
extrude "Extrude12" [no effect]
sketch "Sketch13" plane through (0, 0, -9.5) normal (0, 0, -1) x (1, 0, 0)
  arc A0 (2.475846, -95.000001) -> (4.475846, -93.000001) centre (2.475846, -93.000001) ccw
  line L0 (4.475846, -93.000001) -> (4.475846, -10.427071)
  line L1 (4.475846, -10.427071) -> (-5.524154, -10.427071)
  line L2 (-5.524154, -10.427071) -> (-5.524154, -97.000001)
  arc A1 (-3.524154, -95.000001) -> (-5.524154, -97.000001) centre (-3.524154, -97.000001) ccw
  line L3 (-3.524154, -95.000001) -> (2.475846, -95.000001)
  circle A2 centre (-1.524154, -18.427071) radius 3
  circle A3 centre (-1.524154, -87.000001) radius 3
  dimension "d76" = 6
  dimension "d78" = 6
  measures "d76" diameter of A2
  measures "d78" diameter of A3
extrude "Extrude13" cut sketch "Sketch13" against normal blind 3 contours A2 picked at (-1.024154, -17.561045) bodies 3
extrude "Extrude14" cut sketch "Sketch13" against normal blind 3 contours A3 picked at (0.242156, -86.501269) bodies 3
sketch "Sketch14" plane through (0, 0, -9.453789) normal (0, 0, -1) x (1, 0, 0)
  arc A0 (283.175761, -93.000001) -> (285.175761, -95.000001) centre (285.175761, -93.000001) ccw
  line L0 (285.175761, -95.000001) -> (291.175761, -95.000001)
  arc A1 (293.175761, -97.000001) -> (291.175761, -95.000001) centre (291.175761, -97.000001) ccw
  line L1 (293.175761, -97.000001) -> (293.175761, -10.048794)
  line L2 (293.175761, -10.048794) -> (283.175761, -10.048794)
  line L3 (283.175761, -10.048794) -> (283.175761, -93.000001)
  circle A2 centre (289.175761, -18.048794) radius 3
  circle A3 centre (289.175761, -87.000001) radius 3
  dimension "d87" = 6
  dimension "d88" = 6
  measures "d87" diameter of A2
  measures "d88" diameter of A3
extrude "Extrude16" cut sketch "Sketch14" against normal blind 3 contours A3 picked at (289.398282, -87.974929) bodies 3
extrude "Extrude15" cut sketch "Sketch14" against normal blind 3 contours A2 picked at (287.712027, -17.368621) bodies 3
hole "Hole1" at (-1.524154, 18.427071, -9.5) direction (0, 0, 1) diameter 2 depth 14 tip angle 180 bodies 2 3
thread "Thread1" "ISO Metric profile 2.0 M2x0.4 6H" major diameter 2.074 minor diameter 1.623 pitch 0.4 angle 60 resizes the face on face at (-1.474308, 19.425828, -4.333333) on bodies 3
hole "Hole2" at (-1.524154, 87.000001, -9.5) direction (0, 0, 1) diameter 2 depth 14 tip angle 180 bodies 2 3
thread "Thread2" "ISO Metric profile 2.0 M2x0.4 6H" major diameter 2.074 minor diameter 1.623 pitch 0.4 angle 60 resizes the face on face at (-0.634282, 86.543791, -2.166667) on bodies 3
hole "Hole3" at (289.175761, 18.048794, -9.453789) direction (0, 0, 1) diameter 2 depth 14 tip angle 180 bodies 2 3
thread "Thread3" "ISO Metric profile 2.0 M2x0.4 6H" major diameter 2.074 minor diameter 1.623 pitch 0.4 angle 60 resizes the face on face at (288.532974, 18.814838, -4.302526) on bodies 3
hole "Hole4" at (289.175761, 87.000001, -9.453789) direction (0, 0, 1) diameter 2 depth 14 tip angle 180 bodies 2 3
thread "Thread4" "ISO Metric profile 2.0 M2x0.4 6H" major diameter 2.074 minor diameter 1.623 pitch 0.4 angle 60 resizes the face on face at (288.532974, 87.766046, -4.302526) on bodies 3
sketch "Sketch15" plane through (0, -0.990159, -8.105239) normal (0, -0.121261, -0.992621) x (1, 0, 0)
  ellipse E0 centre (-3.524154, -98.718644) end of major axis (-3.524154, -96.703775) minor radius 2 (-3.524154, -96.703775) -> (-5.524154, -98.718644) ccw
  line L0 (-5.524154, -98.718644) -> (-5.524154, -104.059794)
  ellipse E1 centre (-3.524154, -104.059794) end of major axis (-3.524154, -106.074662) minor radius 2 (-5.524154, -104.059794) -> (-3.524154, -106.074662) ccw
  line L1 (-3.524154, -106.074662) -> (291.175761, -106.074662)
  ellipse E2 centre (291.175761, -104.059794) end of major axis (291.175761, -106.074662) minor radius 2 (291.175761, -106.074662) -> (293.175761, -104.059794) ccw
  line L2 (293.175761, -104.059794) -> (293.175761, -98.718644)
  ellipse E3 centre (291.175761, -98.718644) end of major axis (291.175761, -96.703775) minor radius 2 (293.175761, -98.718644) -> (291.175761, -96.703775) ccw
  line L3 (291.175761, -96.703775) -> (285.175761, -96.703775)
  ellipse E4 centre (285.175761, -94.688907) end of major axis (285.175761, -96.703775) minor radius 2 (283.175761, -94.688907) -> (285.175761, -96.703775) ccw
  line L4 (283.175761, -94.688907) -> (283.175761, -11.121019)
  line L5 (283.175761, -11.121019) -> (293.175761, -11.121019)
  line L6 (293.175761, -11.121019) -> (293.175761, 0.914661)
  ellipse E5 centre (291.175761, 0.914661) end of major axis (291.175761, 2.929529) minor radius 2 (293.175761, 0.914661) -> (291.175761, 2.929529) ccw
  line L7 (291.175761, 2.929529) -> (-3.524154, 2.929529)
  ellipse E6 centre (-3.524154, 0.914661) end of major axis (-3.524154, 2.929529) minor radius 2 (-3.524154, 2.929529) -> (-5.524154, 0.914661) ccw
  line L8 (-5.524154, 0.914661) -> (-5.524154, -11.502108)
  line L9 (-5.524154, -11.502108) -> (4.475846, -11.502108)
  line L10 (4.475846, -11.502108) -> (4.475846, -94.688907)
  ellipse E7 centre (2.475846, -94.688907) end of major axis (2.475846, -96.703775) minor radius 2 (2.475846, -96.703775) -> (4.475846, -94.688907) ccw
  line L11 (2.475846, -96.703775) -> (-3.524154, -96.703775)
  circle A0 centre (4.475846, -5.293724) radius 4
  dimension "d106" = 8
  measures "d106" diameter of A0
extrude "Extrude17" cut sketch "Sketch15" against normal blind 0.5 contours A0 picked at (2.590378, -4.483892) bodies 3
sketch "Sketch16" plane through (0, -0.990159, -8.105239) normal (0, -0.121261, -0.992621) x (1, 0, 0)
  circle A0 centre (4.475846, -5.293724) radius 4
  ellipse E0 centre (-3.524154, -98.718644) end of major axis (-3.524154, -96.703775) minor radius 2 (-3.524154, -96.703775) -> (-5.524154, -98.718644) ccw
  line L0 (-5.524154, -98.718644) -> (-5.524154, -104.059794)
  ellipse E1 centre (-3.524154, -104.059794) end of major axis (-3.524154, -106.074662) minor radius 2 (-5.524154, -104.059794) -> (-3.524154, -106.074662) ccw
  line L1 (-3.524154, -106.074662) -> (291.175761, -106.074662)
  ellipse E2 centre (291.175761, -104.059794) end of major axis (291.175761, -106.074662) minor radius 2 (291.175761, -106.074662) -> (293.175761, -104.059794) ccw
  line L2 (293.175761, -104.059794) -> (293.175761, -98.718644)
  ellipse E3 centre (291.175761, -98.718644) end of major axis (291.175761, -96.703775) minor radius 2 (293.175761, -98.718644) -> (291.175761, -96.703775) ccw
  line L3 (291.175761, -96.703775) -> (285.175761, -96.703775)
  ellipse E4 centre (285.175761, -94.688907) end of major axis (285.175761, -96.703775) minor radius 2 (283.175761, -94.688907) -> (285.175761, -96.703775) ccw
  line L4 (283.175761, -94.688907) -> (283.175761, -11.121019)
  line L5 (283.175761, -11.121019) -> (293.175761, -11.121019)
  line L6 (293.175761, -11.121019) -> (293.175761, 0.914661)
  ellipse E5 centre (291.175761, 0.914661) end of major axis (291.175761, 2.929529) minor radius 2 (293.175761, 0.914661) -> (291.175761, 2.929529) ccw
  line L7 (291.175761, 2.929529) -> (-3.524154, 2.929529)
  ellipse E6 centre (-3.524154, 0.914661) end of major axis (-3.524154, 2.929529) minor radius 2 (-3.524154, 2.929529) -> (-5.524154, 0.914661) ccw
  line L8 (-5.524154, 0.914661) -> (-5.524154, -11.502108)
  line L9 (-5.524154, -11.502108) -> (4.475846, -11.502108)
  line L10 (4.475846, -11.502108) -> (4.475846, -94.688907)
  ellipse E7 centre (2.475846, -94.688907) end of major axis (2.475846, -96.703775) minor radius 2 (2.475846, -96.703775) -> (4.475846, -94.688907) ccw
  line L11 (2.475846, -96.703775) -> (-3.524154, -96.703775)
  circle A1 centre (283.175761, -5.103179) radius 4
  circle A2 centre (283.175761, -101.389219) radius 4
  circle A3 centre (4.475846, -101.389219) radius 4
  dimension "d110" = 8
  dimension "d112" = 8
  dimension "d114" = 8
  measures "d110" diameter of A1
  measures "d112" diameter of A2
  measures "d114" diameter of A3